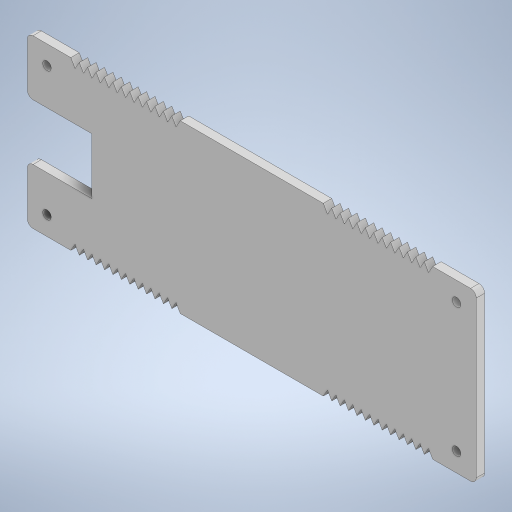
# Autodesk Inventor part: BatteryCarrier SlideRail ToothMountPlate
Saved by Autodesk Inventor 2023 (Build 270158000, 158)
## iProperties
Created: 2023-01-18
Part Number: BatteryCarrier SlideRail ToothMountPlate
Material: Generic
Document SubType Name: Modeling
Designer: Administrator
Density: 1 g/cm^3
Appearance: Default
Author: Administrator
Autodesk Inventor part; units mm, degrees
ref_plane "YZ Plane" through (0, 0, 0) normal (1, 0, 0) x (0, 1, 0)
ref_plane "XZ Plane" through (0, 0, 0) normal (0, 1, 0) x (-1, 0, 0)
ref_plane "XY Plane" through (0, 0, 0) normal (0, 0, 1) x (1, 0, 0)
sketch "Sketch1" plane through (0, 0, 0) normal (0, 0, 1) x (1, 0, 0)
  line L0 (0, 0) -> (146, 0) construction
  line L1 (146, 0) -> (146, 46) construction
  line L2 (146, 46) -> (0, 46) construction
  line L3 (0, 46) -> (0, 0) construction
  circle A0 centre (0, 46) radius 1.5
  circle A1 centre (0, 0) radius 1.5
  circle A2 centre (146, 0) radius 1.5
  circle A3 centre (146, 46) radius 1.5
  line L4 (0, 0) -> (146, 46) construction
  line L5 (-7, -6.75) -> (153, -6.75)
  line L6 (153, -6.75) -> (153, 52.75)
  line L7 (153, 52.75) -> (-7, 52.75)
  line L8 (-7, 52.75) -> (-7, -6.75)
  line L9 (-7, -6.75) -> (153, 52.75) construction
  line L10 (153, -6.75) -> (-7, 52.75) construction
  line L11 (73, 23) -> (93, 23) construction
  line L12 (73, 23) -> (73, 43) construction
  line L13 (116.5, -6.75) -> (118, -4.1519)
  line L14 (116.5, -6.75) -> (119.5, -6.75) construction
  line L15 (118, -4.1519) -> (119.5, -6.75)
  line L16 (26.5, -6.75) -> (28, -4.1519)
  line L17 (26.5, -6.75) -> (29.5, -6.75) construction
  line L18 (28, -4.1519) -> (29.5, -6.75)
  line L19 (26.5, -6.75) -> (29.5, -6.75)
  line L20 (119.5, -6.75) -> (116.5, -6.75)
  line L21 (-7, 33) -> (16, 33)
  line L22 (16, 33) -> (16, 13)
  line L23 (16, 13) -> (-7, 13)
  line L24 (-7, 13) -> (-7, 33)
  dimension "d0" = 146
  dimension "d1" = 46
  dimension "d2" = 3
  dimension "d3" = 3
  dimension "d4" = 3
  dimension "d5" = 3
  dimension "d6" = 160
  dimension "d7" = 59.5
  dimension "d8" = 20
  dimension "d9" = 20
  dimension "d10" = 3
  dimension "d11" = 60
  dimension "d12" = 3
  dimension "d13" = 60
  dimension "d14" = 3
  dimension "d15" = 60
  dimension "d16" = 3
  dimension "d17" = 60
  dimension "d18" = 90
  dimension "d19" = 35
  dimension "d30" = 23
  dimension "d31" = 20
  dimension "d32" = 19.75
  constraints: 50 end point, 6 horizontal, 6 parallel, 4 centre point, 4 coincident, 4 perpendicular, 3 midpoint, 2 collinear, 2 equal length, 1 point on line
  measures "d0" distance of L2.end L1.end
  measures "d1" distance of L1.end L0.end
  measures "d2" diameter of A0
  measures "d3" diameter of A1
  measures "d4" diameter of A2
  measures "d5" diameter of A3
  measures "d6" distance of L7.end L6.end
  measures "d7" distance of L6.end L5.end
  measures "d8" distance of L11.start L11.end
  measures "d9" distance of L11.start L12.end
  measures "d10" distance of L13.start L13.end
  measures "d11" angle of L14 L13
  measures "d12" distance of L13.end L15.end
  measures "d13" angle of L13 L15
  measures "d14" distance of L16.start L16.end
  measures "d15" angle of L17 L16
  measures "d16" distance of L16.end L18.end
  measures "d17" angle of L16 L18
  measures "d18" distance of L13.end L16.end
  measures "d19" distance from line of L6 L13.end
  measures "d30" distance of L22.end L23.end
  measures "d31" distance of L21.end L22.end
  measures "d32" distance between parallel lines of L7 L21
extrude "Extrusion1" add sketch "Sketch1" along normal blind 3 contours L8 L23 L22 L21 L7 L6 L5 L15 L13 L18 L16
extrude "Extrusion2" cut sketch "Sketch1" along normal blind 10 contours L16 L18 L5 | L13 L15 L5
pattern_linear "Rectangular Pattern1" count 7 spacing 3 along (1, 0, 0) of "Extrusion2"
pattern_linear "Rectangular Pattern2" count 7 spacing 3 along (-1, 0, 0) of "Extrusion2"
ref_plane "Work Plane1" through (-7, 23, 0) normal (0, 1, 0) x (1, 0, 0)
mirror "Mirror1" about plane through (-7, 23, 0) normal (0, 1, 0) of "Extrusion2", "Rectangular Pattern1", "Rectangular Pattern2"
fillet "Fillet1" radius 2 6 edges at (-7, 52.75, 1.5) (-7, 13, 1.5) (-7, -6.75, 1.5) (-7, 33, 1.5) (153, 52.75, 1.5) (153, -6.75, 1.5)
equation "\"d19\" = -0.5 * d18 + 0.5 * d6"
equation "\"d32\" = -0.5 * d31 + 0.5 * d7"
body "Solid1"
